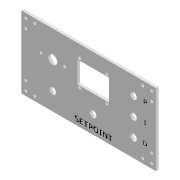
# Autodesk Inventor part: base_2
Saved by Autodesk Inventor 2022 (Build 260153000, 153)
## iProperties
Created: 2022-11-06
Part Number: base_2
Material: Genérico
Document SubType Name: Modeling
Designer: Jorge
Density: 1 g/cm^3
Appearance: Valor por defecto
Author: Jorge
Autodesk Inventor part; units mm, degrees
note: some values were not read from the file. Chosen so that the rebuilt part matches the saved one: direction of "Repujado1".
ref_plane "YZ Plane" through (0, 0, 0) normal (1, 0, 0) x (0, 1, 0)
ref_plane "XZ Plane" through (0, 0, 0) normal (0, 1, 0) x (-1, 0, 0)
ref_plane "XY Plane" through (0, 0, 0) normal (0, 0, 1) x (1, 0, 0)
sketch "Boceto1" plane through (0, 0, 0) normal (0, 0, 1) x (1, 0, 0)
  line L0 (0, 0) -> (150, 0)
  line L1 (150, 0) -> (150, 80)
  line L2 (150, 80) -> (0, 80)
  line L3 (0, 80) -> (0, 0)
  dimension "d0" = 150
  dimension "d1" = 80
  constraints: 8 end point, 2 parallel, 1 horizontal, 1 perpendicular
  measures "d0" distance of L2.end L1.end
  measures "d1" distance of L1.end L0.end
extrude "Extrusión1" add sketch "Boceto1" along normal blind 3
sketch "Boceto2" plane through (0, 0, 3) normal (0, 0, 1) x (1, 0, 0)
  line L0 (150, 0) -> (150, 80) construction
  line L1 (150, 80) -> (0, 80) construction
  line L2 (0, 80) -> (0, 0) construction
  line L3 (0, 0) -> (150, 0) construction
  line L4 (0, 80) -> (0, 0) construction
  line L5 (150, 0) -> (150, 80) construction
  line L6 (150, 80) -> (0, 80) construction
  line L7 (0, 0) -> (150, 0) construction
  line L8 (125, 80) -> (125, 0) construction
  line L9 (35, 80) -> (35, 0) construction
  line L10 (80, 80) -> (80, 0) construction
  line L11 (0, 20) -> (150, 20) construction
  line L12 (0, 40) -> (150, 40) construction
  line L13 (0, 60) -> (150, 60) construction
  circle A0 centre (125, 60) radius 3.6
  circle A1 centre (125, 40) radius 3.6
  circle A2 centre (125, 20) radius 3.6
  line L14 (0, 40) -> (150, 40) construction
  circle A3 centre (80, 20) radius 3.6
  circle A4 centre (35, 20) radius 3.6
  line L15 (62.5, 64) -> (97.5, 64)
  line L16 (97.5, 64) -> (97.5, 40)
  line L17 (97.5, 40) -> (62.5, 40)
  line L18 (62.5, 40) -> (62.5, 64)
  circle A5 centre (35, 50) radius 5
  dimension "d4" = 7.2
  dimension "d5" = 7.2
  dimension "d6" = 7.2
  dimension "d7" = 20
  dimension "d8" = 20
  dimension "d9" = 20
  dimension "d10" = 25
  dimension "d13" = 7.2
  dimension "d14" = 45
  dimension "d15" = 7.2
  dimension "d16" = 35
  dimension "d17" = 35
  dimension "d18" = 24
  dimension "d19" = 17.5
  dimension "d20" = 40
  dimension "d21" = 10
  dimension "d22" = 10
  constraints: 22 end point, 20 point on line, 7 perpendicular, 6 centre point, 5 midpoint, 2 parallel, 1 horizontal
  measures "d4" diameter of A0
  measures "d5" diameter of A1
  measures "d6" diameter of A2
  measures "d7" distance between parallel lines of L12 L13
  measures "d8" distance between parallel lines of L11 L12
  measures "d9" distance between parallel lines of L14 L11
  measures "d10" distance between parallel lines of L5 L8
  measures "d13" diameter of A3
  measures "d14" distance between parallel lines of L8 L10
  measures "d15" diameter of A4
  measures "d16" distance between parallel lines of L9 L2
  measures "d17" distance of L15.start L15.end
  measures "d18" distance of L15.end L16.end
  measures "d19" distance between parallel lines of L10 L18
  measures "d20" distance between parallel lines of L7 L17
  measures "d21" diameter of A5
  measures "d22" distance from line of L13 A5.centre
extrude "Extrusión2" cut sketch "Boceto2" against normal blind 10
sketch "Boceto3" plane through (0, 0, 3) normal (0, 0, 1) x (1, 0, 0)
  circle A0 centre (125, 20) radius 3.6 construction
  circle A1 centre (125, 60) radius 3.6 construction
  circle A2 centre (125, 40) radius 3.6 construction
  circle A3 centre (35, 50) radius 5 construction
  line L0 (97.5, 64) -> (97.5, 40) construction
  line L1 (97.5, 40) -> (62.5, 40) construction
  line L2 (62.5, 40) -> (62.5, 64) construction
  line L3 (62.5, 64) -> (97.5, 64) construction
  circle A4 centre (80, 20) radius 3.6 construction
  circle A5 centre (35, 20) radius 3.6 construction
  line L4 (150, 0) -> (150, 80) construction
  line L5 (150, 80) -> (0, 80) construction
  line L6 (0, 80) -> (0, 0) construction
  line L7 (0, 0) -> (150, 0) construction
  line L8 (150, 80) -> (0, 80) construction
  line L9 (64.775, 80) -> (64.775, 0) construction
  line L10 (0, 0) -> (150, 0) construction
  line L11 (95.225, 80) -> (95.225, 0) construction
  line L12 (0, 80) -> (0, 0) construction
  line L13 (0, 66.2) -> (150, 66.2) construction
  line L14 (0, 37.8) -> (150, 37.8) construction
  circle A6 centre (95.225, 66.2) radius 1.6
  circle A7 centre (64.775, 66.2) radius 1.6
  circle A8 centre (64.775, 37.8) radius 1.6
  circle A9 centre (95.225, 37.8) radius 1.6
  line L15 (97.5, 64) -> (62.5, 64) construction
  line L16 (80, 64) -> (80, 40) construction
  line L17 (62.5, 40) -> (97.5, 40) construction
  line L18 (62.5, 40) -> (62.5, 64) construction
  line L19 (62.5, 52) -> (97.5, 52) construction
  line L20 (97.5, 64) -> (97.5, 40) construction
  dimension "d25" = 3.2
  dimension "d26" = 3.2
  dimension "d27" = 3.2
  dimension "d28" = 3.2
  dimension "d29" = 30.45
  dimension "d32" = 15.225
  dimension "d41" = 28.4
  dimension "d42" = 14.2
  constraints: 16 point on line, 12 end point, 4 centre point, 4 midpoint, 3 perpendicular, 1 vertical
  measures "d25" diameter of A6
  measures "d26" diameter of A7
  measures "d27" diameter of A8
  measures "d28" diameter of A9
  measures "d29" distance between parallel lines of L11 L9
  measures "d32" distance between parallel lines of L16 L9
  measures "d41" distance between parallel lines of L14 L13
  measures "d42" distance between parallel lines of L19 L13
extrude "Extrusión3" cut sketch "Boceto3" against normal blind 10
sketch "Boceto4" plane through (0, 0, 3) normal (0, 0, 1) x (1, 0, 0)
  circle A0 centre (35, 50) radius 5 construction
  line L0 (21.9, 50) -> (35, 50) construction
  line L1 (35, 50) -> (48.1, 50) construction
  circle A1 centre (21.9, 50) radius 1.6
  circle A2 centre (48.1, 50) radius 1.6
  point P0 (0, 0)
  dimension "d35" = 3.2
  dimension "d36" = 3.2
  dimension "d37" = 26.2
  dimension "d38" = 13.1
  constraints: 4 end point, 2 centre point, 2 coincident, 2 horizontal
  measures "d35" diameter of A1
  measures "d36" diameter of A2
  measures "d37" distance of L1.end L0.start
  measures "d38" distance of L0.end L0.start
extrude "Extrusión4" cut sketch "Boceto4" against normal through all
sketch "Boceto5" plane through (0, 0, 3) normal (0, 0, 1) x (1, 0, 0)
  circle A0 centre (21.9, 50) radius 1.6 construction
  circle A1 centre (48.1, 50) radius 1.6 construction
  circle A2 centre (64.775, 37.8) radius 1.6 construction
  circle A3 centre (64.775, 66.2) radius 1.6 construction
  circle A4 centre (95.225, 66.2) radius 1.6 construction
  circle A5 centre (95.225, 37.8) radius 1.6 construction
  circle A6 centre (125, 20) radius 3.6 construction
  circle A7 centre (125, 60) radius 3.6 construction
  circle A8 centre (125, 40) radius 3.6 construction
  circle A9 centre (35, 50) radius 5 construction
  line L0 (97.5, 64) -> (97.5, 40) construction
  line L1 (97.5, 40) -> (62.5, 40) construction
  line L2 (62.5, 40) -> (62.5, 64) construction
  line L3 (62.5, 64) -> (97.5, 64) construction
  circle A10 centre (80, 20) radius 3.6 construction
  circle A11 centre (35, 20) radius 3.6 construction
  line L4 (150, 0) -> (150, 80) construction
  line L5 (150, 80) -> (0, 80) construction
  line L6 (0, 80) -> (0, 0) construction
  line L7 (0, 0) -> (150, 0) construction
  circle A12 centre (125, 60) radius 3.6 construction
  line L8 (125, 60) -> (150, 60) construction
  line L9 (150, 0) -> (150, 80) construction
  circle A13 centre (125, 40) radius 3.6 construction
  line L10 (125, 40) -> (150, 40) construction
  circle A14 centre (125, 20) radius 3.6 construction
  line L11 (125, 20) -> (150, 20) construction
  circle A15 centre (80, 20) radius 3.6 construction
  line L12 (80, 20) -> (80, 0) construction
  line L13 (0, 0) -> (150, 0) construction
  line L14 (134.0212, 42.7124) -> (140.9788, 42.7124) construction
  line L15 (140.9788, 42.7124) -> (140.9788, 37.2876) construction
  line L16 (140.9788, 37.2876) -> (134.0212, 37.2876) construction
  line L17 (134.0212, 37.2876) -> (134.0212, 42.7124) construction
  line L18 (134.0212, 40) -> (140.9788, 40) construction
  line L19 (137.5, 42.7124) -> (137.5, 37.2876) construction
  line L20 (134.0212, 22.7124) -> (140.9788, 22.7124) construction
  line L21 (140.9788, 22.7124) -> (140.9788, 17.2876) construction
  line L22 (140.9788, 17.2876) -> (134.0212, 17.2876) construction
  line L23 (134.0212, 17.2876) -> (134.0212, 22.7124) construction
  line L24 (134.0212, 20) -> (140.9788, 20) construction
  line L25 (137.5, 22.7124) -> (137.5, 17.2876) construction
  line L26 (134.0212, 62.7124) -> (140.9788, 62.7124) construction
  line L27 (140.9788, 62.7124) -> (140.9788, 57.2876) construction
  line L28 (140.9788, 57.2876) -> (134.0212, 57.2876) construction
  line L29 (134.0212, 57.2876) -> (134.0212, 62.7124) construction
  line L30 (134.0212, 60) -> (140.9788, 60) construction
  line L31 (137.5, 62.7124) -> (137.5, 57.2876) construction
  line L32 (60.3816, 9.5307) -> (99.6184, 9.5307) construction
  line L33 (99.6184, 9.5307) -> (99.6184, 2.4693) construction
  line L34 (99.6184, 2.4693) -> (60.3816, 2.4693) construction
  line L35 (60.3816, 2.4693) -> (60.3816, 9.5307) construction
  line L36 (60.3816, 6) -> (99.6184, 6) construction
  line L37 (80, 9.5307) -> (80, 2.4693) construction
  spline S0 degree 2 poles (61.2075, 2.893) (60.517, 2.893) (59.4765, 3.1605) (59.0292, 3.3549) knots 0 0 0 1 2 2 2
  line L38 (59.0292, 3.3549) -> (59.0292, 4.7844)
  line L39 (59.0292, 4.7844) -> (59.1653, 4.7844)
  spline S1 degree 2 poles (59.1653, 4.7844) (59.6175, 4.4003) (60.7018, 3.987) (61.2123, 3.987) knots 0 0 0 1 2 2 2
  spline S2 degree 2 poles (61.2123, 3.987) (61.3436, 3.987) (61.7666, 4.0454) (61.893, 4.1037) knots 0 0 0 1 2 2 2
  spline S3 degree 2 poles (61.893, 4.1037) (62.0486, 4.1718) (62.2674, 4.4198) (62.2674, 4.6191) knots 0 0 0 1 2 2 2
  spline S4 degree 2 poles (62.2674, 4.6191) (62.2674, 4.8476) (61.9125, 5.1297) (61.6694, 5.1929) knots 0 0 0 1 2 2 2
  spline S5 degree 2 poles (61.6694, 5.1929) (61.363, 5.2755) (60.6677, 5.4165) (60.3614, 5.5235) knots 0 0 0 1 2 2 2
  spline S6 degree 2 poles (60.3614, 5.5235) (59.6661, 5.7666) (59.0632, 6.5981) (59.0632, 7.2204) knots 0 0 0 1 2 2 2
  spline S7 degree 2 poles (59.0632, 7.2204) (59.0632, 8.0616) (60.4878, 9.107) (61.5575, 9.107) knots 0 0 0 1 2 2 2
  spline S8 degree 2 poles (61.5575, 9.107) (62.0924, 9.107) (63.1523, 8.8882) (63.5705, 8.7034) knots 0 0 0 1 2 2 2
  line L40 (63.5705, 8.7034) -> (63.5705, 7.3323)
  line L41 (63.5705, 7.3323) -> (63.4392, 7.3323)
  spline S9 degree 2 poles (63.4392, 7.3323) (63.1037, 7.6191) (62.141, 8.013) (61.6353, 8.013) knots 0 0 0 1 2 2 2
  spline S10 degree 2 poles (61.6353, 8.013) (61.436, 8.013) (61.1248, 7.9546) (60.9498, 7.8768) knots 0 0 0 1 2 2 2
  spline S11 degree 2 poles (60.9498, 7.8768) (60.8088, 7.8136) (60.6045, 7.5608) (60.6045, 7.4052) knots 0 0 0 1 2 2 2
  spline S12 degree 2 poles (60.6045, 7.4052) (60.6045, 7.1718) (60.9303, 6.9044) (61.3971, 6.7974) knots 0 0 0 1 2 2 2
  spline S13 degree 2 poles (61.3971, 6.7974) (61.6985, 6.7293) (62.2577, 6.5981) (62.5786, 6.4862) knots 0 0 0 1 2 2 2
  spline S14 degree 2 poles (62.5786, 6.4862) (63.201, 6.2577) (63.8088, 5.4992) (63.8088, 4.8768) knots 0 0 0 1 2 2 2
  spline S15 degree 2 poles (63.8088, 4.8768) (63.8088, 3.9822) (62.4036, 2.893) (61.2075, 2.893) knots 0 0 0 1 2 2 2
  line L42 (64.5818, 3) -> (64.5818, 9)
  line L43 (64.5818, 9) -> (68.637, 9)
  line L44 (68.637, 9) -> (68.637, 7.8574)
  line L45 (68.637, 7.8574) -> (66.0794, 7.8574)
  line L46 (66.0794, 7.8574) -> (66.0794, 6.8023)
  line L47 (66.0794, 6.8023) -> (68.4376, 6.8023)
  line L48 (68.4376, 6.8023) -> (68.4376, 5.6596)
  line L49 (68.4376, 5.6596) -> (66.0794, 5.6596)
  line L50 (66.0794, 5.6596) -> (66.0794, 4.1426)
  line L51 (66.0794, 4.1426) -> (68.637, 4.1426)
  line L52 (68.637, 4.1426) -> (68.637, 3)
  line L53 (68.637, 3) -> (64.5818, 3)
  line L54 (70.8104, 3) -> (70.8104, 7.8574)
  line L55 (70.8104, 7.8574) -> (69.0357, 7.8574)
  line L56 (69.0357, 7.8574) -> (69.0357, 9)
  line L57 (69.0357, 9) -> (74.0924, 9)
  line L58 (74.0924, 9) -> (74.0924, 7.8574)
  line L59 (74.0924, 7.8574) -> (72.3177, 7.8574)
  line L60 (72.3177, 7.8574) -> (72.3177, 3)
  line L61 (72.3177, 3) -> (70.8104, 3)
  spline S16 degree 2 poles (79.3241, 7.1086) (79.3241, 6.6904) (79.0567, 5.9319) (78.8088, 5.6791) knots 0 0 0 1 2 2 2
  spline S17 degree 2 poles (78.8088, 5.6791) (78.658, 5.5186) (78.2885, 5.2561) (78.0697, 5.1637) knots 0 0 0 1 2 2 2
  spline S18 degree 2 poles (78.0697, 5.1637) (77.846, 5.0713) (77.3258, 4.9643) (77.0049, 4.9643) knots 0 0 0 1 2 2 2
  line L62 (77.0049, 4.9643) -> (76.2172, 4.9643)
  line L63 (76.2172, 4.9643) -> (76.2172, 3)
  line L64 (76.2172, 3) -> (74.7099, 3)
  line L65 (74.7099, 3) -> (74.7099, 9)
  line L66 (74.7099, 9) -> (77.0389, 9)
  spline S19 degree 2 poles (77.0389, 9) (77.5543, 9) (78.3079, 8.8104) (78.6143, 8.6062) knots 0 0 0 1 2 2 2
  spline S20 degree 2 poles (78.6143, 8.6062) (78.9546, 8.3776) (79.3241, 7.6288) (79.3241, 7.1086) knots 0 0 0 1 2 2 2
  spline S21 degree 2 poles (77.778, 7.0697) (77.778, 7.3274) (77.5348, 7.6921) (77.3695, 7.7601) knots 0 0 0 1 2 2 2
  spline S22 degree 2 poles (77.3695, 7.7601) (77.1556, 7.8525) (76.7666, 7.8817) (76.4311, 7.8817) knots 0 0 0 1 2 2 2
  line L67 (76.4311, 7.8817) -> (76.2172, 7.8817)
  line L68 (76.2172, 7.8817) -> (76.2172, 6.0827)
  line L69 (76.2172, 6.0827) -> (76.3241, 6.0827)
  spline S23 degree 2 poles (76.3241, 6.0827) (76.5332, 6.0827) (76.9125, 6.0924) (77.0535, 6.1167) knots 0 0 0 1 2 2 2
  spline S24 degree 2 poles (77.0535, 6.1167) (77.175, 6.1361) (77.4425, 6.2528) (77.5154, 6.3258) knots 0 0 0 1 2 2 2
  spline S25 degree 2 poles (77.5154, 6.3258) (77.671, 6.4716) (77.778, 6.7974) (77.778, 7.0697) knots 0 0 0 1 2 2 2
  spline S26 degree 2 poles (85.5916, 6) (85.5916, 4.5413) (84.0357, 2.8736) (82.684, 2.8736) knots 0 0 0 1 2 2 2
  spline S27 degree 2 poles (82.684, 2.8736) (81.3274, 2.8736) (79.7812, 4.5608) (79.7812, 6) knots 0 0 0 1 2 2 2
  spline S28 degree 2 poles (79.7812, 6) (79.7812, 7.4441) (81.3274, 9.1264) (82.684, 9.1264) knots 0 0 0 1 2 2 2
  spline S29 degree 2 poles (82.684, 9.1264) (84.0357, 9.1264) (85.5916, 7.4538) (85.5916, 6) knots 0 0 0 1 2 2 2
  spline S30 degree 2 poles (84.0357, 6) (84.0357, 6.5397) (83.8169, 7.2934) (83.6272, 7.5316) knots 0 0 0 1 2 2 2
  spline S31 degree 2 poles (83.6272, 7.5316) (83.4376, 7.7796) (82.9514, 7.9935) (82.6888, 7.9935) knots 0 0 0 1 2 2 2
  spline S32 degree 2 poles (82.6888, 7.9935) (82.4117, 7.9935) (81.9595, 7.7942) (81.7504, 7.5413) knots 0 0 0 1 2 2 2
  spline S33 degree 2 poles (81.7504, 7.5413) (81.5656, 7.3079) (81.3371, 6.5348) (81.3371, 6) knots 0 0 0 1 2 2 2
  spline S34 degree 2 poles (81.3371, 6) (81.3371, 5.4457) (81.5559, 4.7164) (81.7455, 4.4684) knots 0 0 0 1 2 2 2
  spline S35 degree 2 poles (81.7455, 4.4684) (81.9352, 4.2204) (82.4263, 4.0065) (82.6888, 4.0065) knots 0 0 0 1 2 2 2
  spline S36 degree 2 poles (82.6888, 4.0065) (82.9562, 4.0065) (83.4522, 4.235) (83.6321, 4.4781) knots 0 0 0 1 2 2 2
  spline S37 degree 2 poles (83.6321, 4.4781) (83.8266, 4.7407) (84.0357, 5.436) (84.0357, 6) knots 0 0 0 1 2 2 2
  line L70 (89.4716, 3) -> (86.2431, 3)
  line L71 (86.2431, 3) -> (86.2431, 4.0454)
  line L72 (86.2431, 4.0454) -> (87.1037, 4.0454)
  line L73 (87.1037, 4.0454) -> (87.1037, 7.9546)
  line L74 (87.1037, 7.9546) -> (86.2431, 7.9546)
  line L75 (86.2431, 7.9546) -> (86.2431, 9)
  line L76 (86.2431, 9) -> (89.4716, 9)
  line L77 (89.4716, 9) -> (89.4716, 7.9546)
  line L78 (89.4716, 7.9546) -> (88.611, 7.9546)
  line L79 (88.611, 7.9546) -> (88.611, 4.0454)
  line L80 (88.611, 4.0454) -> (89.4716, 4.0454)
  line L81 (89.4716, 4.0454) -> (89.4716, 3)
  line L82 (95.6126, 3) -> (94.1637, 3)
  line L83 (94.1637, 3) -> (91.8493, 7.1815)
  line L84 (91.8493, 7.1815) -> (91.8493, 3)
  line L85 (91.8493, 3) -> (90.4733, 3)
  line L86 (90.4733, 3) -> (90.4733, 9)
  line L87 (90.4733, 9) -> (92.3209, 9)
  line L88 (92.3209, 9) -> (94.2366, 5.5624)
  line L89 (94.2366, 5.5624) -> (94.2366, 9)
  line L90 (94.2366, 9) -> (95.6126, 9)
  line L91 (95.6126, 9) -> (95.6126, 3)
  line L92 (97.9854, 3) -> (97.9854, 7.8574)
  line L93 (97.9854, 7.8574) -> (96.2107, 7.8574)
  line L94 (96.2107, 7.8574) -> (96.2107, 9)
  line L95 (96.2107, 9) -> (101.2674, 9)
  line L96 (101.2674, 9) -> (101.2674, 7.8574)
  line L97 (101.2674, 7.8574) -> (99.4927, 7.8574)
  line L98 (99.4927, 7.8574) -> (99.4927, 3)
  line L99 (99.4927, 3) -> (97.9854, 3)
  spline S38 degree 2 poles (139.8764, 20.2084) (139.8764, 19.5074) (139.2646, 18.4053) (138.7986, 18.1095) knots 0 0 0 1 2 2 2
  spline S39 degree 2 poles (138.7986, 18.1095) (138.4096, 17.8583) (137.4939, 17.7124) (136.9793, 17.7124) knots 0 0 0 1 2 2 2
  line L100 (136.9793, 17.7124) -> (135.4153, 17.7124)
  line L101 (135.4153, 17.7124) -> (135.4153, 22.7124)
  line L102 (135.4153, 22.7124) -> (136.9631, 22.7124)
  spline S40 degree 2 poles (136.9631, 22.7124) (137.4899, 22.7124) (138.4096, 22.5787) (138.8148, 22.3194) knots 0 0 0 1 2 2 2
  spline S41 degree 2 poles (138.8148, 22.3194) (139.3051, 22.0034) (139.8764, 20.9337) (139.8764, 20.2084) knots 0 0 0 1 2 2 2
  spline S42 degree 2 poles (138.5879, 20.2165) (138.5879, 20.7108) (138.2476, 21.4158) (137.8991, 21.6144) knots 0 0 0 1 2 2 2
  spline S43 degree 2 poles (137.8991, 21.6144) (137.6438, 21.7521) (137.0847, 21.7805) (136.6957, 21.7805) knots 0 0 0 1 2 2 2
  line L103 (136.6957, 21.7805) -> (136.6714, 21.7805)
  line L104 (136.6714, 21.7805) -> (136.6714, 18.6484)
  line L105 (136.6714, 18.6484) -> (136.6957, 18.6484)
  spline S44 degree 2 poles (136.6957, 18.6484) (137.1171, 18.6484) (137.6965, 18.6768) (137.9599, 18.8429) knots 0 0 0 1 2 2 2
  spline S45 degree 2 poles (137.9599, 18.8429) (138.2678, 19.0374) (138.5879, 19.7222) (138.5879, 20.2165) knots 0 0 0 1 2 2 2
  line L106 (138.8452, 37.7124) -> (136.1548, 37.7124)
  line L107 (136.1548, 37.7124) -> (136.1548, 38.5836)
  line L108 (136.1548, 38.5836) -> (136.872, 38.5836)
  line L109 (136.872, 38.5836) -> (136.872, 41.8413)
  line L110 (136.872, 41.8413) -> (136.1548, 41.8413)
  line L111 (136.1548, 41.8413) -> (136.1548, 42.7124)
  line L112 (136.1548, 42.7124) -> (138.8452, 42.7124)
  line L113 (138.8452, 42.7124) -> (138.8452, 41.8413)
  line L114 (138.8452, 41.8413) -> (138.128, 41.8413)
  line L115 (138.128, 41.8413) -> (138.128, 38.5836)
  line L116 (138.128, 38.5836) -> (138.8452, 38.5836)
  line L117 (138.8452, 38.5836) -> (138.8452, 37.7124)
  spline S46 degree 2 poles (139.6049, 61.1363) (139.6049, 60.7878) (139.3821, 60.1557) (139.1754, 59.945) knots 0 0 0 1 2 2 2
  spline S47 degree 2 poles (139.1754, 59.945) (139.0498, 59.8113) (138.7419, 59.5925) (138.5596, 59.5155) knots 0 0 0 1 2 2 2
  spline S48 degree 2 poles (138.5596, 59.5155) (138.3732, 59.4385) (137.9396, 59.3494) (137.6722, 59.3494) knots 0 0 0 1 2 2 2
  line L118 (137.6722, 59.3494) -> (137.0158, 59.3494)
  line L119 (137.0158, 59.3494) -> (137.0158, 57.7124)
  line L120 (137.0158, 57.7124) -> (135.7597, 57.7124)
  line L121 (135.7597, 57.7124) -> (135.7597, 62.7124)
  line L122 (135.7597, 62.7124) -> (137.7006, 62.7124)
  spline S49 degree 2 poles (137.7006, 62.7124) (138.1301, 62.7124) (138.7581, 62.5544) (139.0134, 62.3842) knots 0 0 0 1 2 2 2
  spline S50 degree 2 poles (139.0134, 62.3842) (139.297, 62.1938) (139.6049, 61.5698) (139.6049, 61.1363) knots 0 0 0 1 2 2 2
  spline S51 degree 2 poles (138.3165, 61.1038) (138.3165, 61.3186) (138.1139, 61.6225) (137.9761, 61.6792) knots 0 0 0 1 2 2 2
  spline S52 degree 2 poles (137.9761, 61.6792) (137.7978, 61.7562) (137.4737, 61.7805) (137.1941, 61.7805) knots 0 0 0 1 2 2 2
  line L123 (137.1941, 61.7805) -> (137.0158, 61.7805)
  line L124 (137.0158, 61.7805) -> (137.0158, 60.2813)
  line L125 (137.0158, 60.2813) -> (137.1049, 60.2813)
  spline S53 degree 2 poles (137.1049, 60.2813) (137.2792, 60.2813) (137.5952, 60.2894) (137.7127, 60.3097) knots 0 0 0 1 2 2 2
  spline S54 degree 2 poles (137.7127, 60.3097) (137.814, 60.3259) (138.0369, 60.4231) (138.0976, 60.4839) knots 0 0 0 1 2 2 2
  spline S55 degree 2 poles (138.0976, 60.4839) (138.2273, 60.6055) (138.3165, 60.8769) (138.3165, 61.1038) knots 0 0 0 1 2 2 2
  point P0 (134.729, 67.5051)
  point P1 (141.6867, 67.5051)
  point P2 (137.5, 60)
  point P3 (137.5, 40)
  point P4 (137.5, 20)
  point P5 (137.5, 40)
  point P6 (137.5, 20)
  point P7 (137.5, 60)
  dimension "d43" = 0
  dimension "d44" = 6
  constraints: 24 end point, 23 midpoint, 3 horizontal, 3 perpendicular, 3 point on line, 8 other
  measures "d43" distance between parallel lines of L12 L37
  measures "d44" distance between parallel lines of L7 L36
emboss "Repujado1" sketch "Boceto5" operation cut depth 0.5 direction (0, 0, -1)
sketch "Boceto6" plane through (0, 0, 3) normal (0, 0, 1) x (1, 0, 0)
  line L0 (150, 0) -> (150, 80) construction
  line L1 (150, 80) -> (0, 80) construction
  line L2 (0, 80) -> (0, 0) construction
  line L3 (0, 0) -> (150, 0) construction
  circle A0 centre (35, 20) radius 3.6 construction
  circle A1 centre (80, 20) radius 3.6 construction
  line L4 (97.5, 64) -> (97.5, 40) construction
  line L5 (97.5, 40) -> (62.5, 40) construction
  line L6 (62.5, 40) -> (62.5, 64) construction
  line L7 (62.5, 64) -> (97.5, 64) construction
  circle A2 centre (35, 50) radius 5 construction
  circle A3 centre (125, 40) radius 3.6 construction
  circle A4 centre (125, 60) radius 3.6 construction
  circle A5 centre (125, 20) radius 3.6 construction
  circle A6 centre (95.225, 37.8) radius 1.6 construction
  circle A7 centre (95.225, 66.2) radius 1.6 construction
  circle A8 centre (64.775, 66.2) radius 1.6 construction
  circle A9 centre (64.775, 37.8) radius 1.6 construction
  circle A10 centre (48.1, 50) radius 1.6 construction
  circle A11 centre (21.9, 50) radius 1.6 construction
  line L8 (137.6722, 59.3494) -> (137.0158, 59.3494) construction
  line L9 (137.0158, 59.3494) -> (137.0158, 57.7124) construction
  line L10 (137.0158, 57.7124) -> (135.7597, 57.7124) construction
  line L11 (135.7597, 62.7124) -> (137.7006, 62.7124) construction
  line L12 (137.7006, 62.7124) -> (139.0134, 62.7124) construction
  line L13 (135.4153, 17.7124) -> (135.4153, 22.7124) construction
  line L14 (135.4153, 22.7124) -> (136.9631, 22.7124) construction
  line L15 (136.9793, 17.7124) -> (135.4153, 17.7124) construction
  line L16 (97.9854, 3) -> (97.9854, 7.8574) construction
  line L17 (97.9854, 7.8574) -> (96.2107, 7.8574) construction
  line L18 (96.2107, 7.8574) -> (96.2107, 9) construction
  line L19 (96.2107, 9) -> (101.2674, 9) construction
  line L20 (101.2674, 9) -> (101.2674, 7.8574) construction
  line L21 (101.2674, 7.8574) -> (99.4927, 7.8574) construction
  line L22 (99.4927, 7.8574) -> (99.4927, 3) construction
  line L23 (99.4927, 3) -> (97.9854, 3) construction
  line L24 (90.4733, 9) -> (92.3209, 9) construction
  line L25 (92.3209, 9) -> (94.2366, 5.5624) construction
  line L26 (94.2366, 5.5624) -> (94.2366, 9) construction
  line L27 (94.2366, 9) -> (95.6126, 9) construction
  line L28 (95.6126, 9) -> (95.6126, 3) construction
  line L29 (95.6126, 3) -> (94.1637, 3) construction
  line L30 (94.1637, 3) -> (91.8493, 7.1815) construction
  line L31 (91.8493, 7.1815) -> (91.8493, 3) construction
  line L32 (91.8493, 3) -> (90.4733, 3) construction
  line L33 (90.4733, 3) -> (90.4733, 9) construction
  line L34 (89.4716, 3) -> (86.2431, 3) construction
  line L35 (86.2431, 3) -> (86.2431, 4.0454) construction
  line L36 (86.2431, 4.0454) -> (87.1037, 4.0454) construction
  line L37 (87.1037, 4.0454) -> (87.1037, 7.9546) construction
  line L38 (87.1037, 7.9546) -> (86.2431, 7.9546) construction
  line L39 (86.2431, 7.9546) -> (86.2431, 9) construction
  line L40 (86.2431, 9) -> (89.4716, 9) construction
  line L41 (89.4716, 9) -> (89.4716, 7.9546) construction
  line L42 (89.4716, 7.9546) -> (88.611, 7.9546) construction
  line L43 (88.611, 7.9546) -> (88.611, 4.0454) construction
  line L44 (88.611, 4.0454) -> (89.4716, 4.0454) construction
  line L45 (89.4716, 4.0454) -> (89.4716, 3) construction
  line L46 (74.0924, 9) -> (74.0924, 7.8574) construction
  line L47 (74.0924, 7.8574) -> (72.3177, 7.8574) construction
  line L48 (72.3177, 7.8574) -> (72.3177, 3) construction
  line L49 (72.3177, 3) -> (70.8104, 3) construction
  line L50 (70.8104, 3) -> (70.8104, 7.8574) construction
  line L51 (70.8104, 7.8574) -> (69.0357, 7.8574) construction
  line L52 (69.0357, 7.8574) -> (69.0357, 9) construction
  line L53 (69.0357, 9) -> (74.0924, 9) construction
  line L54 (63.5705, 8.7034) -> (63.5705, 7.3323) construction
  line L55 (63.5705, 7.3323) -> (63.4392, 7.3323) construction
  line L56 (59.0292, 3.3549) -> (59.0292, 4.7844) construction
  line L57 (59.0292, 4.7844) -> (59.1653, 4.7844) construction
  line L58 (77.0049, 4.9643) -> (76.2172, 4.9643) construction
  line L59 (76.2172, 4.9643) -> (76.2172, 3) construction
  line L60 (76.2172, 3) -> (74.7099, 3) construction
  line L61 (74.7099, 9) -> (77.0389, 9) construction
  line L62 (77.0389, 9) -> (78.6143, 9) construction
  line L63 (68.4376, 6.8023) -> (68.4376, 5.6596) construction
  line L64 (68.4376, 5.6596) -> (66.0794, 5.6596) construction
  line L65 (66.0794, 5.6596) -> (66.0794, 4.1426) construction
  line L66 (66.0794, 4.1426) -> (68.637, 4.1426) construction
  line L67 (68.637, 4.1426) -> (68.637, 3) construction
  line L68 (68.637, 3) -> (64.5818, 3) construction
  line L69 (64.5818, 3) -> (64.5818, 9) construction
  line L70 (64.5818, 9) -> (68.637, 9) construction
  line L71 (68.637, 9) -> (68.637, 7.8574) construction
  line L72 (68.637, 7.8574) -> (66.0794, 7.8574) construction
  line L73 (66.0794, 7.8574) -> (66.0794, 6.8023) construction
  line L74 (66.0794, 6.8023) -> (68.4376, 6.8023) construction
  line L75 (136.1548, 42.7124) -> (138.8452, 42.7124) construction
  line L76 (138.8452, 42.7124) -> (138.8452, 41.8413) construction
  line L77 (138.8452, 41.8413) -> (138.128, 41.8413) construction
  line L78 (138.128, 41.8413) -> (138.128, 38.5836) construction
  line L79 (138.128, 38.5836) -> (138.8452, 38.5836) construction
  line L80 (138.8452, 38.5836) -> (138.8452, 37.7124) construction
  line L81 (138.8452, 37.7124) -> (136.1548, 37.7124) construction
  line L82 (136.1548, 37.7124) -> (136.1548, 38.5836) construction
  line L83 (136.1548, 38.5836) -> (136.872, 38.5836) construction
  line L84 (136.872, 38.5836) -> (136.872, 41.8413) construction
  line L85 (136.872, 41.8413) -> (136.1548, 41.8413) construction
  line L86 (136.1548, 41.8413) -> (136.1548, 42.7124) construction
  line L87 (0, 80) -> (0, 0) construction
  line L88 (0, 75) -> (150, 75) construction
  line L89 (150, 80) -> (0, 80) construction
  line L90 (5, 80) -> (5, 0) construction
  line L91 (0, 0) -> (150, 0) construction
  line L92 (145, 80) -> (145, 0) construction
  line L93 (0, 5) -> (150, 5) construction
  line L94 (0, 65) -> (150, 65) construction
  line L95 (150, 0) -> (150, 80) construction
  line L96 (15, 80) -> (15, 0) construction
  line L97 (0, 15) -> (150, 15) construction
  line L98 (135, 80) -> (135, 0) construction
  circle A12 centre (5, 75) radius 1.6
  circle A13 centre (5, 65) radius 1.6
  circle A14 centre (15, 75) radius 1.6
  circle A15 centre (5, 15) radius 1.6
  circle A16 centre (5, 5) radius 1.6
  circle A17 centre (15, 5) radius 1.6
  circle A18 centre (135, 5) radius 1.6
  circle A19 centre (145, 5) radius 1.6
  circle A20 centre (145, 15) radius 1.6
  circle A21 centre (135, 75) radius 1.6
  circle A22 centre (145, 75) radius 1.6
  circle A23 centre (145, 65) radius 1.6
  line L99 (135.7597, 57.7124) -> (135.7597, 62.7124) projected
  line L100 (74.7099, 3) -> (74.7099, 9) projected
  dimension "d47" = 5
  dimension "d48" = 5
  dimension "d49" = 5
  dimension "d50" = 5
  dimension "d51" = 10
  dimension "d52" = 10
  dimension "d53" = 10
  dimension "d54" = 10
  dimension "d55" = 3.2
  dimension "d56" = 3.2
  dimension "d57" = 3.2
  dimension "d58" = 3.2
  dimension "d59" = 3.2
  dimension "d60" = 3.2
  dimension "d61" = 3.2
  dimension "d62" = 3.2
  dimension "d63" = 3.2
  dimension "d64" = 3.2
  dimension "d65" = 3.2
  dimension "d66" = 3.2
  constraints: 40 point on line, 16 end point, 12 centre point, 7 perpendicular, 1 parallel, 32 other
  measures "d47" distance between parallel lines of L0 L92
  measures "d48" distance between parallel lines of L3 L93
  measures "d49" distance between parallel lines of L1 L88
  measures "d50" distance between parallel lines of L2 L90
  measures "d51" distance between parallel lines of L88 L94
  measures "d52" distance between parallel lines of L90 L96
  measures "d53" distance between parallel lines of L92 L98
  measures "d54" distance between parallel lines of L93 L97
  measures "d55" diameter of A12
  measures "d56" diameter of A13
  measures "d57" diameter of A14
  measures "d58" diameter of A15
  measures "d59" diameter of A16
  measures "d60" diameter of A17
  measures "d61" diameter of A18
  measures "d62" diameter of A19
  measures "d63" diameter of A20
  measures "d64" diameter of A21
  measures "d65" diameter of A22
  measures "d66" diameter of A23
extrude "Extrusión5" cut sketch "Boceto6" against normal through all
equation "\"d5\" = d4"
equation "\"d6\" = d4"
equation "\"d9\" = d8"
equation "\"d15\" = d4"
equation "\"d19\" = 0.5 * d17"
equation "\"d32\" = 0.5 * d29"
equation "\"d42\" = 0.5 * d41"
equation "\"d38\" = 0.5 * d37"
